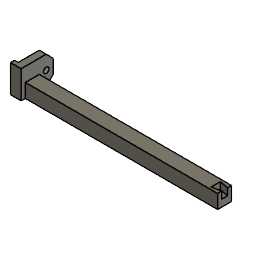
_NewBackstopB - PLA.2799a766-dff8-46e4-9405-490c11756fb7 (Autodesk Fusion 360 design; units mm, degrees)
Autodesk Fusion 360 part; units mm, degrees
sketch "Sketch1" plane through (0, 0, 0) normal (0, 1, 0) x (1, 0, 0)
  line L0 (0, 0) -> (-25, 0)
  line L1 (-25, 0) -> (-25, -5)
  line L2 (-25, -5) -> (5, -5)
  line L3 (0, 0) -> (0, 10)
  line L4 (0, 10) -> (5, 10)
  line L5 (5, 10) -> (5, -5)
  line L6 (-25, 0) -> (-245, 0)
  line L7 (-245, 0) -> (-245, -5)
  line L8 (-245, -5) -> (-25, -5)
  line L9 (-25, 0) -> (-140, 0)
  line L10 (-140, 0) -> (-140, 27.0089)
  line L11 (-270, 10) -> (-275, 10)
  line L12 (-270, 0) -> (-270, 10)
  line L13 (-275, 10) -> (-275, -5)
  line L14 (-270, 0) -> (-245, 0)
  line L15 (-245, -5) -> (-275, -5)
  line L16 (-245, 0) -> (-245, -5)
  point P0 (-270, 0)
  dimension "d1" = 25
  dimension "d2" = 5
  dimension "d3" = 30
  dimension "d4" = 10
  dimension "d5" = 5
  dimension "d6" = 220
  dimension "d7" = 5
  dimension "d8" = 115
  constraint coincident L0.start L3.start
  constraint horizontal L0
  constraint perpendicular L0 L1
  constraint perpendicular L1 L2
  constraint perpendicular L0 L3
  constraint perpendicular L3 L4
  constraint perpendicular L1 L6
  constraint perpendicular L6 L7
  constraint perpendicular L1 L9
  constraint perpendicular L6 L10
  measures "d1" distance of L0.start L0.end
  measures "d2" distance of L0.end L1.end
  measures "d3" distance of L1.end L2.end
  measures "d4" distance of L0.start L3.end
  measures "d5" distance of L3.end L4.end
  measures "d6" distance of L0.end L6.end
  measures "d7" distance of L6.end L7.end
  measures "d8" distance of L0.end L9.end
extrude "Extrude1" add sketch "Sketch1" along normal blind 10
extrude "Extrude2" add sketch "Sketch1" along normal blind 20 contours L0 L1 L2 L3 L4 L5 | L7 L11 L12 L13 L14 L15 L16
sketch "Sketch2" plane through (5, 0, 0) normal (1, 0, 0) x (0, 0, -1)
  line L0 (-5, 0) -> (10, 0)
  line L1 (10, 0) -> (10, 20)
  line L2 (10, 20) -> (-5, 20)
  line L3 (-5, 20) -> (-5, 0)
sketch "Sketch3" plane through (0, 0, 0) normal (-1, 0, 0) x (0, 0, 1)
  line L0 (-10, 0) -> (0, 0)
  line L1 (0, 0) -> (0, 20)
  line L2 (0, 20) -> (-10, 20)
  line L3 (-10, 20) -> (-10, 0)
  line L4 (-10, 0) -> (-5, 0)
  line L5 (-5, 0) -> (-5, 10)
  circle A0 centre (-5, 10) radius 2.5
  dimension "d13" = 5
  dimension "d14" = 10
  dimension "d15" = 5
  constraint coincident L0.start L3.end
  constraint midpoint L0 L4.end
  constraint perpendicular L4 L5
  constraint coincident L5.end A0.centre
  measures "d13" distance of L0.start L4.end
  measures "d14" distance of L4.end L5.end
  measures "d15" diameter of A0
extrude "Extrude3" cut sketch "Sketch3" along normal mid plane 662 contours A0
chamfer "Chamfer1" distance 5 angle 45 4 edges at (2.5, 20, -10) (2.5, 0, -10) (-272.5, 20, -10) (-272.5, 0, -10)
sketch "Sketch5" plane through (0, 10, 0) normal (0, 1, 0) x (-1, 0, 0)
  line L0 (25, 5) -> (25, 0)
  line L1 (25, 0) -> (245, 0)
  line L2 (245, 0) -> (245, 5)
  line L3 (245, 5) -> (25, 5)
  line L4 (245, 0) -> (135, 0)
  dimension "d30" = 110
  constraint coincident L1.end L2.start
  constraint perpendicular L0 L4
  measures "d30" distance of L1.end L4.end
sketch "Sketch6" plane through (0, 0, 5) normal (0, 0, 1) x (1, 0, 0)
  line L0 (-25, 10) -> (-245, 10)
  line L1 (-245, 10) -> (-245, 20)
  line L2 (-245, 20) -> (-275, 20)
  line L3 (-275, 20) -> (-275, 0)
  line L4 (-275, 0) -> (5, 0)
  line L5 (5, 0) -> (5, 20)
  line L6 (5, 20) -> (-25, 20)
  line L7 (-25, 20) -> (-25, 10)
extrude "Extrude5" add 1 faces at (-265, 10, 5) along direction (0, 0, 1) blind 5
sketch "Sketch7" plane through (0, 10, 0) normal (0, 1, 0) x (-1, 0, 0)
  line L0 (25, 10) -> (25, 0)
  line L1 (25, 0) -> (245, 0)
  line L2 (245, 0) -> (245, 10)
  line L3 (245, 10) -> (25, 10)
  line L4 (245, 0) -> (135, 0)
  line L5 (138.7555, 1.7499) -> (132.3542, 2.8786)
  line L6 (138.7555, 8.2499) -> (132.3542, 7.1212)
  line L7 (132.3542, 2.8786) -> (132.3904, 0)
  line L8 (138.7555, 8.2499) -> (138.7555, 1.7499)
  line L9 (132.3542, 7.1212) -> (132.3542, 10)
  line L10 (138.7555, 1.7499) -> (141.0619, 1.7499) construction
  line L11 (138.7555, 8.2499) -> (141.0619, 8.2499) construction
  line L12 (25, 0) -> (245, 0)
  line L13 (128.521, 0) -> (128.521, 5)
  line L14 (270, -5) -> (275, -5)
  line L15 (275, -5) -> (275, 10)
  line L16 (275, 10) -> (245, 10)
  line L17 (245, 10) -> (245, 0)
  line L18 (245, 0) -> (270, 0)
  line L19 (270, 0) -> (270, -5)
  point P0 (132.1074, 10.0354)
  point P1 (138.7555, 4.9999)
  dimension "d33" = 110
  dimension "d34" = 6.5
  dimension "d35" = 170
  dimension "d36" = 6.5
  dimension "d37" = 170
  dimension "d38" = 6.5
  dimension "d41" = 5
  constraint coincident L1.end L2.start
  constraint perpendicular L2 L4
  constraint vertical L8
  constraint horizontal L11
  constraint horizontal L10
  constraint vertical L9
  constraint coincident L5.start L8.end
  constraint coincident L7.end L12
  constraint coincident L3 L9.end
  constraint coincident L12 L13.start
  constraint perpendicular L12 L13
  constraint midpoint L8 P1
  constraint equal L7 L9
  measures "d33" distance of L1.end L4.end
  measures "d34" distance of L6.start L5.start
  measures "d35" angle of L6 L11
  measures "d36" distance of L6.end L6.start
  measures "d37" angle of L5 L10
  measures "d38" distance of L5.start L5.end
  measures "d41" distance of L13.start L13.end
extrude "Extrude8" cut sketch "Sketch7" against normal blind 5 contours L0 L1 L3 L5 L6 L7 L8 L9 L12
sketch "Sketch10" plane through (0, 0, 5) normal (0, 0, 1) x (1, 0, 0)
  line L0 (-138.7555, 5) -> (-132.3542, 5)
  line L1 (-132.3542, 5) -> (-25, 5)
  line L2 (-25, 5) -> (-132.3904, 5)
  line L3 (-132.3542, 5) -> (-138.7555, 5)
  line L4 (-275, 0) -> (-270, 0)
  line L5 (-270, 0) -> (0, 0)
  line L6 (0, 0) -> (5, 0)
  line L7 (5, 0) -> (-275, 0)
  line L8 (-25, 5) -> (-132.3542, 5)
  line L9 (-132.3904, 5) -> (-132.3542, 5)
  line L10 (-132.3542, 10) -> (-132.3904, 10)
  line L11 (-132.3542, 10) -> (-132.3904, 10)
  point P0 (-132.3542, 10)
sketch "Sketch11" plane through (0, 5, 0) normal (0, 1, 0) x (-1, 0, 0)
  line L0 (138.7555, 8.2499) -> (132.3542, 7.1212)
  line L1 (132.3542, 7.1212) -> (132.3542, 10)
  line L2 (132.3542, 10) -> (25, 10)
  line L3 (25, 10) -> (25, 0)
  line L4 (25, 0) -> (132.3904, 0)
  line L5 (132.3904, 0) -> (132.3542, 2.8786)
  line L6 (132.3542, 2.8786) -> (138.7555, 1.7499)
  line L7 (138.7555, 1.7499) -> (138.7555, 8.2499)
  line L8 (132.3904, 0) -> (132.3904, 13.7938)
  line L9 (132.3904, 13.7938) -> (-13.9928, 13.7938)
  line L10 (-13.9928, 13.7938) -> (-13.9928, -23.8644)
  line L11 (-13.9928, -23.8644) -> (132.3904, -21.0994)
  line L12 (132.3904, -21.0994) -> (132.3904, 0)
  constraint coincident L4.end L5.start
  constraint perpendicular L2 L8
  constraint perpendicular L8 L9
  constraint perpendicular L9 L10
  constraint perpendicular L4 L12
extrude "Extrude9" cut sketch "Sketch11" along normal mid plane 40 contours L0 L1 L2 L3 L4 L5 L6 L8 | L0 L1 L2 L3 L4 L8 L9 L10 L11 L12 | L5 L6 L8
sketch "Sketch12" plane through (0, 20, 0) normal (0, 1, 0) x (-1, 0, 0)
  line L0 (270, -5) -> (275, -5)
  line L1 (275, -5) -> (275, 10)
  line L2 (275, 10) -> (245, 10)
  line L3 (270, 0) -> (245, 0)
  line L4 (245, 0) -> (245, 10)
  line L5 (245, 10) -> (270, 10)
  line L6 (270, 10) -> (270, 0)
  constraint horizontal L3
  constraint vertical L4
  constraint horizontal L5
  constraint vertical L6
  constraint coincident L2.end L4.end
extrude "Extrude10" cut sketch "Sketch12" against normal blind 10
sketch "Sketch13" plane through (-270, 0, 0) normal (1, 0, 0) x (0, 0, -1)
  circle A0 centre (5, 10) radius 2.5
  line L0 (5, 0) -> (10, 5)
  line L1 (10, 5) -> (10, 15)
  line L2 (10, 15) -> (5, 20)
  line L3 (5, 20) -> (0, 20)
  line L4 (0, 20) -> (-10, 20)
  line L5 (-10, 20) -> (-10, 10)
  line L6 (-10, 10) -> (0, 10)
  line L7 (0, 10) -> (0, 0)
  line L8 (0, 0) -> (5, 0)
sketch "Sketch14" plane through (0, 0, 10) normal (0, 0, 1) x (1, 0, 0)
  line L0 (-132.3904, 10) -> (-270, 10)
  line L1 (-270, 10) -> (-270, 20)
  line L2 (-270, 20) -> (-275, 20)
  line L3 (-275, 20) -> (-275, 0)
  line L4 (-275, 0) -> (-132.3904, 0)
  line L5 (-132.3904, 0) -> (-132.3904, 10)
  line L6 (-270, 20) -> (-277.675, 20)
  line L7 (-277.675, 20) -> (-277.675, 0)
  line L8 (-277.675, 0) -> (-270, 0)
  line L9 (-270, 0) -> (-270, 20)
  dimension "d54" = 7.675
  constraint horizontal L6
  constraint vertical L7
  constraint horizontal L8
  constraint vertical L9
  constraint coincident L1.end L2.start
  measures "d54" distance of L1.end L6.end
extrude "Extrude11" add sketch "Sketch14" along normal blind 3 contours L1 L2 L3 L4 L6 L8 L9 | L3 L6 L7 L8
sketch "Sketch15" plane through (-270, 0, 0) normal (1, 0, 0) x (0, 0, -1)
  circle A0 centre (5, 10) radius 2.5
  circle A1 centre (5, 10) radius 2
  dimension "d57" = 5
  dimension "d58" = 4
  constraint concentric A0 A1
  measures "d57" diameter of A0
  measures "d58" diameter of A1
extrude "Extrude12" add sketch "Sketch15" against normal blind 5
extrude "Extrude6" [suppressed]
sketch "Sketch8" plane through (0, 5, 0) normal (0, 1, 0) x (-1, 0, 0)
  line L0 (138.2622, 7.9923) -> (138.2622, 1.9923)
  line L1 (138.2622, 1.9923) -> (132.3533, 3.0342)
  line L2 (132.3533, 3.0342) -> (132.3533, 0)
  line L3 (132.3533, 0) -> (245, 0)
  line L4 (245, 0) -> (245, 10)
  line L5 (245, 10) -> (132.3533, 10)
  line L6 (132.3533, 10) -> (132.3533, 6.9504)
  line L7 (132.3533, 6.9504) -> (138.2622, 7.9923)
  line L8 (245, 5) -> (25, 5)
  line L9 (270, -5) -> (275, -5)
  line L10 (275, -5) -> (275, 10)
  line L11 (275, 10) -> (245, 10)
  line L12 (245, 10) -> (245, 0)
  line L13 (245, 0) -> (270, 0)
  line L14 (270, 0) -> (270, -5)
  line L15 (275, -10) -> (275, -5)
  line L16 (275, -5) -> (270, -5)
  line L17 (270, -5) -> (270, -10)
  line L18 (270, -10) -> (275, -10)
sketch "Sketch9" plane through (0, 20, 0) normal (0, 1, 0) x (-1, 0, 0)
  line L0 (270, -5) -> (275, -5)
  line L1 (275, -5) -> (275, 10)
  line L2 (275, 10) -> (245, 10)
  line L3 (245, 10) -> (245, 0)
  line L4 (245, 0) -> (270, 0)
  line L5 (270, 0) -> (270, -5)
  line L6 (275, -10) -> (275, -5)
  line L7 (275, -5) -> (270, -5)
  line L8 (270, -5) -> (270, -10)
  line L9 (270, -10) -> (275, -10)
  line L10 (138.2622, 7.9923) -> (138.2622, 1.9923)
  line L11 (138.2622, 1.9923) -> (132.3533, 3.0342)
  line L12 (132.3533, 3.0342) -> (132.3533, 0)
  line L13 (132.3533, 0) -> (245, 0)
  line L14 (245, 0) -> (245, 10)
  line L15 (245, 10) -> (132.3533, 10)
  line L16 (132.3533, 10) -> (132.3533, 6.9504)
  line L17 (132.3533, 6.9504) -> (138.2622, 7.9923)
  line L18 (138.2622, 1.9923) -> (138.2622, -2.244)
  line L19 (138.2622, -2.244) -> (138.2622, 11)
  constraint coincident L10.end L11.start
  constraint perpendicular L13 L18
  constraint perpendicular L15 L19
extrude "Extrude7" [suppressed]
equation "d54 = 5 mm + ( 25.4 / 8 ) * 1 mm - 0.5 mm"
